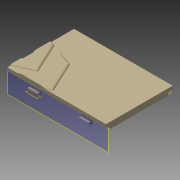
# Autodesk Inventor part: Deckel
Saved by Autodesk Inventor 2014 (Build 180170000, 170)
## iProperties
Created: 2016-07-27
Part Number: Deckel
Material: Generisch
Document SubType Name: Modeling
Designer: cem
Density: 1 g/cm^3
Appearance: Beige
Author: cem
Autodesk Inventor part; units mm, degrees
ref_plane "YZ Plane" through (0, 0, 0) normal (1, 0, 0) x (0, 1, 0)
ref_plane "XZ Plane" through (0, 0, 0) normal (0, 1, 0) x (-1, 0, 0)
ref_plane "XY Plane" through (0, 0, 0) normal (0, 0, 1) x (1, 0, 0)
sketch "SkizzeDeckel" plane through (0, 0, 0) normal (0, 0, 1) x (1, 0, 0)
  line L0 (-30.24, 0) -> (30.24, 0) projected
  line L1 (0, -20.44) -> (0, 20.44) projected
  line L2 (21.6, -14.6) -> (-21.6, -14.6) projected
  line L3 (-21.6, 14.6) -> (21.6, 14.6)
  line L4 (21.6, 14.6) -> (21.6, -14.6)
  line L5 (21.6, -14.6) -> (-21.6, -14.6)
  line L6 (-21.6, -14.6) -> (-21.6, 14.6)
  line L7 (-21.6, -14.6) -> (-21.6, -9.7) projected
  point P0 (0, 0)
  constraints: 8 end point, 2 collinear, 2 parallel, 1 horizontal, 1 perpendicular, 2 other
extrude "Deckel" add sketch "SkizzeDeckel" along normal blind 1.5
sketch "SkizzeStecker" plane through (0, 0, 0) normal (0, 0, -1) x (-1, 0, 0)
  line L0 (-21.6, 14.6) -> (-21.6, -14.6) projected
  line L1 (21.6, -14.6) -> (21.6, 14.6) projected
  line L2 (-20.1, -12.7) -> (-20.1, 12.7) projected
  line L3 (-21.6, -12.7) -> (-20.1, -12.7) projected
  line L4 (-21.6, 12.7) -> (-21.6, -12.7) projected
  line L5 (-21.6, 12.7) -> (-20.1, 12.7) projected
  line L6 (20.1, 9.7) -> (20.1, -9.7) projected
  line L7 (21.6, 9.7) -> (20.1, 9.7) projected
  line L8 (21.6, -9.7) -> (21.6, 9.7) projected
  line L9 (21.6, -9.7) -> (20.1, -9.7) projected
  line L10 (-21.6, -12.65) -> (-20.1, -12.65)
  line L11 (-20.1, -12.65) -> (-20.1, 12.65)
  line L12 (-20.1, 12.65) -> (-21.6, 12.65)
  line L13 (-21.6, 12.65) -> (-21.6, -12.65)
  line L14 (30.24, 0) -> (-30.24, 0) projected
  line L15 (21.6, 9.65) -> (20.1, 9.65)
  line L16 (20.1, 9.65) -> (20.1, -9.65)
  line L17 (20.1, -9.65) -> (21.6, -9.65)
  line L18 (21.6, -9.65) -> (21.6, 9.65)
  point P0 (0, 0)
  dimension "d2" = 0.05
  dimension "d4" = 0.05
  constraints: 16 end point, 5 parallel, 3 collinear, 2 horizontal, 2 perpendicular, 2 other
  measures "d2" distance between parallel lines of L5 L12
  measures "d4" distance between parallel lines of L15 L7
ref_plane "EbeneStecker" through (17.7, 4.9, -1.2) normal (0, 0, 1) x (1, 0, 0)
extrude "Stecker" add sketch "SkizzeStecker" along normal up to surface (1.2 mm away) contours L12 L2 L14 L0 | L14 L2 L10 L0 | L17 L6 L14 L1 | L14 L6 L15 L1
sketch "SkizzeLippe" plane through (0, 0, 0) normal (0, 0, -1) x (-1, 0, 0)
  line L0 (30.24, 0) -> (-30.24, 0) projected
  line L1 (0, -20.44) -> (0, 20.44) projected
  line L2 (-20.75, 13.75) -> (20.75, 13.75)
  line L3 (20.75, 13.75) -> (20.75, -13.75)
  line L4 (20.75, -13.75) -> (-20.75, -13.75)
  line L5 (-20.75, -13.75) -> (-20.75, 13.75)
  line L6 (-20.8, -12.7) -> (-20.8, -13.8) projected
  line L7 (-20.8, -13.8) -> (20.8, -13.8) projected
  line L8 (20.8, 9.7) -> (20.8, 13.8) projected
  line L9 (20.8, 13.8) -> (7.5, 13.8) projected
  point P0 (0, 0)
  dimension "d7" = 0.05
  dimension "d8" = 0.05
  constraints: 8 end point, 2 parallel, 1 horizontal, 1 perpendicular, 2 other
  measures "d7" distance between parallel lines of L8 L3
  measures "d8" distance between parallel lines of L9 L2
ref_plane "LippeEbene" through (0, 0, -0.55) normal (0, 0, 1) x (1, 0, 0)
extrude "Lippe" add sketch "SkizzeLippe" along normal up to surface (0.55 mm away)
sketch "SkizzeSchnapperarm" plane through (20.75, -13.75, -0.55) normal (0, 0, -1) x (-1, 0, 0)
  line L0 (34.15, 0.65) -> (29.65, 0.65) projected
  line L1 (29.7, 0.7) -> (34.1, 0.7)
  line L2 (34.1, 0.7) -> (34.1, 2.2)
  line L3 (34.1, 2.2) -> (29.7, 2.2)
  line L4 (29.7, 2.2) -> (29.7, 0.7)
  line L5 (29.65, -0.85) -> (29.65, 0.65) projected
  line L6 (34.15, -0.85) -> (34.15, 0.65) projected
  line L7 (31.9, -1.277) -> (31.9, 1.312) construction
  point P0 (20.75, 13.75)
  point P1 (31.9, 0.65)
  dimension "d11" = 0.05
  dimension "d12" = 1.5
  dimension "d13" = 0.05
  constraints: 10 end point, 3 parallel, 1 horizontal, 1 midpoint, 1 perpendicular, 1 point on line, 1 other
  measures "d11" distance between parallel lines of L0 L1
  measures "d12" distance between parallel lines of L1 L3
  measures "d13" distance between parallel lines of L4 L5
ref_plane "EbeneSchnapper" through (-8.9, -14.55, -3.85) normal (0, 0, 1) x (1, 0, 0)
extrude "Schnapperarm" add sketch "SkizzeSchnapperarm" along normal up to surface (3.3 mm away)
sketch "SkizzeSchnapper" plane through (-13.35, -13.05, -0.55) normal (0, -1, 0) x (1, 0, 0)
  line L0 (4.4, -3.3) -> (0, -3.3) projected
  line L1 (4.4, 0) -> (4.4, -3.3) projected
  line L2 (-0.05, -1.85) -> (4.45, -1.85) projected
  line L3 (-0.05, -3.45) -> (-0.05, -1.85) projected
  line L4 (4.45, -3.45) -> (-0.05, -3.45) projected
  line L5 (4.45, -1.85) -> (4.45, -3.45) projected
  line L6 (0, -3.3) -> (4.4, -3.3)
  line L7 (4.4, -3.3) -> (4.4, -1.9)
  line L8 (4.4, -1.9) -> (0, -1.9)
  line L9 (0, -1.9) -> (0, -3.3)
  point P0 (13.35, 0.55)
  dimension "d16" = 0.05
  constraints: 8 end point, 2 parallel, 1 horizontal, 1 perpendicular, 1 point on line
  measures "d16" distance between parallel lines of L2 L8
ref_plane "EbeneSchnapperTiefe2" through (-20.1, -13.9, -8.8) normal (0, 1, 0) x (1, 0, 0)
extrude "Schnapper" add sketch "SkizzeSchnapper" along normal up to surface (0.85 mm away) contours L0 L9 L8 L1
chamfer "FaseSchnapper" distance 1.2 distance2 1.1 1 edges at (-11.15, -13.9, -3.85) measured on face at (-11.15, -13.4, -3.85)
draft "FlächenverjüngungSchnapper" angle 12 pull direction (0, 0, -1) fixed plane through (-2.9833, 3.5833, -0.55) normal (0, 0, -1) faces at (-11.8833, -11.55, -1.65)
mirror "SpiegelnSchnapper1" about plane through (0, 0, 0) normal (0, 1, 0) of "Schnapperarm", "Schnapper", "FaseSchnapper", "FlächenverjüngungSchnapper"
mirror "SpiegelnSchnapper2" about plane through (0, 0, 0) normal (1, 0, 0) of "Schnapperarm", "Schnapper", "FaseSchnapper", "FlächenverjüngungSchnapper", "SpiegelnSchnapper1"
sketch "Skizze6" plane through (0, 0, 0) normal (0, 0, -1) x (-1, 0, 0)
  line L0 (21.6, 14.6) -> (-21.6, 14.6)
  line L1 (7.5, 13.8) -> (7.5, 14.6)
  line L2 (-1, 14.6) -> (-1, 13.8)
  line L3 (-1, 13.1) -> (-1, 13.8)
  line L4 (7.5, 13.8) -> (7.5, 13.1)
  line L5 (0.5, 13.1) -> (-1, 13.1)
  line L6 (0.5, 13.1) -> (6, 13.1)
  line L7 (7.5, 13.1) -> (6, 13.1)
  line L8 (-0.95, 13.1) -> (7.45, 13.1)
  line L9 (7.45, 13.1) -> (7.45, 14.6)
  line L10 (7.45, 14.6) -> (-0.95, 14.6)
  line L11 (-0.95, 14.6) -> (-0.95, 13.1)
  line L12 (3.25, 12.1908) -> (3.25, 15.4162) construction
  point P0 (0, 0)
  point P1 (3.25, 13.1)
extrude "USB" add sketch "Skizze6" along normal blind 2 contours L9 L7 L6 L5 L11 L0
sketch "Skizze8" plane through (0, 0, 1.5) normal (0, 0, 1) x (1, 0, 0)
  line L0 (-21.6, 14.6) -> (-21.6, -14.6) projected
  line L1 (-8.9554, 0.1816) -> (-2.6161, -13.4131)
  line L2 (-8.9554, 0.1816) -> (6.0446, 0.1816) construction
  line L3 (-15.6, 2.6) -> (-9.2607, -10.9946)
  line L4 (-9.2607, -10.9946) -> (-20.1364, -16.066)
  line L5 (-15.6, 2.6) -> (-0.6, 2.6) construction
  line L6 (-15.6, 2.6) -> (-8.9554, 0.1816)
  line L7 (-21.6, -14.6) -> (21.6, -14.6) projected
  line L8 (21.6, 14.6) -> (-21.6, 14.6) projected
  line L9 (-20.1364, -16.066) -> (-18.0233, -20.5976)
  line L10 (-2.6161, -13.4131) -> (-18.0233, -20.5976)
  line L11 (-19.5868, 4.0511) -> (-13.2475, -9.5435)
  line L12 (-26.2314, 6.4695) -> (-19.8921, -7.1251)
  line L13 (-19.8921, -7.1251) -> (-30.7678, -12.1965)
  line L14 (-26.2314, 6.4695) -> (-19.5868, 4.0511)
  line L15 (-30.7678, -12.1965) -> (-28.6547, -16.7281)
  line L16 (-13.2475, -9.5435) -> (-28.6547, -16.7281)
  line L17 (-5.1615, -14.6) -> (-16.9925, -14.6)
  line L18 (-21.6, 4.7838) -> (-21.6, -3.4626)
  line L19 (-21.6, -7.9215) -> (-21.6, -13.4384)
  point P0 (0, 0)
  dimension "d28" = 65
  dimension "d32" = 65
  dimension "d37" = 5
  dimension "d38" = 15
  dimension "d39" = 12
  dimension "d40" = 5
  dimension "d41" = 6
  dimension "d42" = 12
  dimension "d43" = 5
  dimension "d44" = 15
  dimension "d45" = 5
  dimension "d46" = 12
  dimension "d48" = 3
  dimension "d49" = 3
  constraints: 34 end point, 12 point on line, 6 perpendicular, 4 equal length, 2 horizontal, 1 parallel
  measures "d28" angle of L1 L2
  measures "d32" angle of L3 L5
  measures "d37" distance between parallel lines of L3 L1
  measures "d38" distance from line of L4 L3.start
  measures "d39" distance between parallel lines of L5 L8
  measures "d40" distance between parallel lines of L10 L4
  measures "d41" distance from line of L3.start L0
  measures "d42" distance between parallel lines of L9 L3
  measures "d43" distance between parallel lines of L12 L11
  measures "d44" distance from line of L13 L14.start
  measures "d45" distance between parallel lines of L16 L13
  measures "d46" distance between parallel lines of L15 L12
  measures "d48" distance between parallel lines of L3 L11
  measures "d49" distance between parallel lines of L4 L16
extrude "Logo" add sketch "Skizze8" along normal blind 0.5 contours L14 L11 L16 L0 L13 L12 | L1 L10 L7 L4 L3 L6
fillet "RundungLogo" radius 1 10 edges at (-12.2777, 1.3908, 2) (-12.4304, -4.1973, 2) (-5.7857, -6.6158, 2) (-13.1266, -12.7973, 2) (-3.8888, -14.0065, 2) (-17.4238, -11.491, 2) (-20.7461, -5.2938, 2) (-20.7461, -7.5233, 2) (-16.4171, -2.7462, 2) (-20.5934, 4.4174, 2)
ref_plane "EbeneStütze" through (17.7, 4.9, -1.45) normal (0, 0, 1) x (1, 0, 0)
sketch "SkizzeStüze" plane through (20.75, -13.75, -0.55) normal (0, 0, -1) x (-1, 0, 0)
  line L0 (6.15, 1.35) -> (-0.05, 1.35) projected
  line L1 (-0.05, 1.35) -> (-0.05, 10.35) projected
  line L2 (-0.05, 10.35) -> (6.15, 10.35) projected
  line L3 (6.15, 10.35) -> (6.15, 1.35) projected
  line L4 (6.15, 11.15) -> (-0.05, 11.15) projected
  line L5 (-0.05, 11.15) -> (-0.05, 26.15) projected
  line L6 (-0.05, 26.15) -> (6.15, 26.15) projected
  line L7 (6.15, 26.15) -> (6.15, 11.15) projected
  line L8 (41.55, 4.35) -> (35.35, 4.35) projected
  line L9 (35.35, 4.35) -> (35.35, 13.35) projected
  line L10 (35.35, 13.35) -> (41.55, 13.35) projected
  line L11 (41.55, 13.35) -> (41.55, 4.35) projected
  line L12 (41.55, 14.15) -> (35.35, 14.15) projected
  line L13 (35.35, 14.15) -> (35.35, 23.15) projected
  line L14 (35.35, 23.15) -> (41.55, 23.15) projected
  line L15 (41.55, 23.15) -> (41.55, 14.15) projected
  line L16 (50.99, 13.75) -> (-9.49, 13.75) projected
  line L17 (20.75, -6.69) -> (20.75, 34.19) projected
  line L18 (3.15, 8.35) -> (38.35, 8.35)
  line L19 (38.35, 8.35) -> (38.35, 6.85)
  line L20 (38.35, 6.85) -> (3.15, 6.85)
  line L21 (3.15, 6.85) -> (3.15, 8.35)
  line L22 (3.15, 19.15) -> (38.35, 19.15)
  line L23 (38.35, 19.15) -> (38.35, 20.65)
  line L24 (38.35, 20.65) -> (3.15, 20.65)
  line L25 (3.15, 20.65) -> (3.15, 19.15)
  point P0 (20.75, 13.75)
  dimension "d53" = 1.5
  dimension "d54" = 3
  dimension "d55" = 2
  constraints: 16 end point, 4 symmetric about line, 2 parallel, 1 horizontal, 1 perpendicular, 1 other
  measures "d53" distance of L18.end L19.end
  measures "d54" distance between parallel lines of L3 L21
  measures "d55" distance between parallel lines of L2 L18
extrude "Extrusion9" add sketch "SkizzeStüze" along normal up to surface (0.9 mm away) contours L20 L21 L18 L3 | L3 L18 L17 L20 | L17 L18 L9 L20 | L9 L18 L19 L20 | L22 L25 L24 L7 | L7 L24 L17 L22 | L17 L24 L13 L22 | L13 L24 L23 L22
